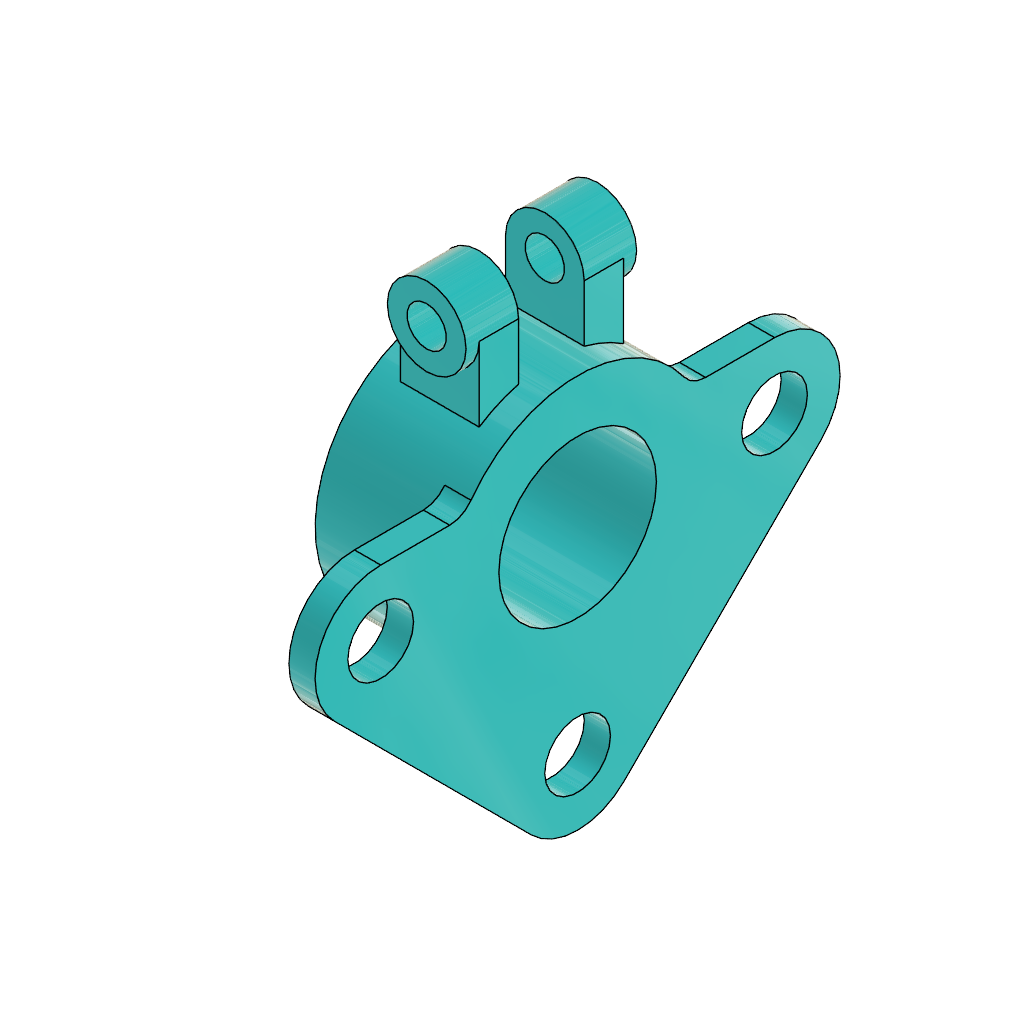
5th pipe clamp (Autodesk Fusion 360 design; units mm, degrees)
part number: 2026-01-13-20-17-19-295
Autodesk Fusion 360 part; units mm, degrees
note: some values were not read from the file. Chosen so that the rebuilt part matches the saved one: which face or edge a step refers to.
cylinder "CylinderPrimitive1" add diameter 100 height 50 placed x (0, 0, -1) y (0, 1, 0) z (1, 0, 0) at (0, 0, 0)
sketch "Sketch2" plane through (50, 0, 0) normal (1, 0, 0) x (0, 1, 0)
  circle A0 centre (0, 0) radius 50
  line L0 (0, 0) -> (125, 0) construction
  line L1 (0, 0) -> (0, -70) construction
  circle A1 centre (75, 0) radius 12.5
  circle A2 centre (75, 0) radius 25
  circle A3 centre (0, -75) radius 12.5
  circle A4 centre (0, -75) radius 25
  circle A5 centre (-75, 0) radius 12.5
  circle A6 centre (-75, 0) radius 25
  line L2 (92.6777, -17.6777) -> (17.6777, -92.6777)
  line L3 (-92.6777, -17.6777) -> (-17.6777, -92.6777)
  line L4 (43.3013, 25) -> (75, 25)
  line L5 (-43.3013, 25) -> (-75, 25)
  line L6 (12.5, 0) -> (27.5, 0)
  line L7 (27.5, 0) -> (27.5, 85)
  line L8 (27.5, 85) -> (12.5, 85)
  line L9 (12.5, 85) -> (12.5, 0)
  dimension "d4" = 25
  dimension "d5" = 50
  dimension "d7" = -180
  dimension "d8" = 15
  dimension "d9" = 85
  dimension "d10" = 12.5
  constraint coincident A0.centre L0.start
  constraint horizontal L0
  constraint perpendicular L0 L1
  constraint coincident L0 A1.centre
  constraint concentric A1 A2
  constraint tangent A0 A2
  constraint coincident A2 L2.start
  constraint tangent A2 L2
  constraint coincident A4 L2.end
  constraint coincident A6 L3.start
  constraint tangent A6 L3
  constraint coincident A4 L3.end
  constraint tangent A4 L3
  constraint tangent A6 L4
  constraint coincident A2 L4.end
  constraint tangent A2 L4
  constraint coincident A0 L4.start
  constraint tangent A4 L2
  constraint symmetric L1 L4.end L5.end
  constraint symmetric L1 L4.start L5.start
  constraint horizontal L6
  constraint vertical L7
  constraint horizontal L8
  constraint vertical L9
  constraint coincident L0 L6.start
  measures "d4" diameter of A1
  measures "d5" diameter of A2
  measures "d8" distance of L6.start L6.end
  measures "d9" distance of L6.end L7.end
  measures "d10" distance of A0.centre L9
extrude "Extrude1" add sketch "Sketch2" against normal blind 10 contours A0 A2 A4 L2 | A0 A2 L4 | A2 | A0 A4 A6 L3 | A4 | A0 A6 L5 | A6
fillet "Fillet1" radius 10 1 edges at (45, -43.3013, 25)
fillet "Fillet2" radius 10 1 edges at (45, 43.3013, 25)
extrude "Extrude2" add sketch "Sketch2" against normal blind 30 from surface at -10 contours A0 L7 L8 L9
fillet "Fillet3" radius 15 2 edges at (40, 20, 85) (10, 20, 85)
cylinder "CylinderPrimitive2" add diameter 30 height 5 placed x (1, 0, 0) y (0, 0, -1) z (0, 1, 0) at (25, 27.5, 70)
hole "Hole1" at (25, 32.5, 70) direction (0, -1, 0) diameter 15 end through all
mirror "Mirror1" about plane through (0, 0, 0) normal (0, 1, 0) of 6 faces at (24.999, 30.8333, 85) (25.001, 22.5, 85) (10, 19.2447, 62.2518) (33.4511, 22.5, 82.3941) (25.6022, 27.5, 46.2086) (25, 12.5, 53.1082)
hole "Hole2" at (0, 0, 0) direction (1, 0, 0) diameter 60 end through all
